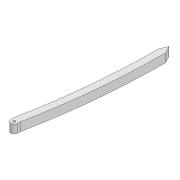
# Autodesk Inventor part: Part_12
Saved by Autodesk Inventor 2022 (Build 260153000, 153)
## iProperties
Created: 2022-05-03
Part Number: Part_12
Material: Generic
Document SubType Name: Modeling
Designer: dell
Density: 1 g/cm^3
Appearance: Default
Author: dell
Autodesk Inventor part; units mm, degrees
ref_plane "YZ Plane" through (0, 0, 0) normal (1, 0, 0) x (0, 1, 0)
ref_plane "XZ Plane" through (0, 0, 0) normal (0, 1, 0) x (-1, 0, 0)
ref_plane "XY Plane" through (0, 0, 0) normal (0, 0, 1) x (1, 0, 0)
sketch "Sketch1" plane through (0, 0, 0) normal (0, 1, 0) x (-1, 0, 0)
  line L0 (0, 0) -> (0, -315.198) construction
  line L1 (-4, 0) -> (-4, -315.198)
  line L2 (4, -315.198) -> (4, 0)
  arc A0 (4, 0) -> (-4, 0) centre (0, 0) ccw
  arc A1 (-4, -315.198) -> (4, -315.198) centre (0, -315.198) ccw
  circle A2 centre (0, 0) radius 1.5
  circle A3 centre (0, -315.198) radius 1.5
  arc A4 (-4, -3) -> (-4, -312.198) centre (780.9198, -157.599) ccw
  arc A5 (4, -3) -> (4, -312.198) centre (788.9198, -157.599) ccw
  point P0 (0, -157.599)
  dimension "d0" = 8
  dimension "d1" = 315.198
  dimension "d2" = 3
  dimension "d3" = 3
  dimension "d24" = 800
  dimension "d25" = 800
  dimension "d26" = 3
  dimension "d27" = 3
  constraints: 8 end point, 8 point on circle, 6 centre point, 4 point on line, 4 tangent, 2 coincident, 2 horizontal alignment, 1 midpoint, 1 parallel, 1 vertical
  measures "d0" diameter of A1
  measures "d1" distance of L0.end L0.start
  measures "d2" diameter of A2
  measures "d3" diameter of A3
  measures "d24" radius of A4
  measures "d25" radius of A5
  measures "d26" vertical distance of L0.end A4.end
  measures "d27" vertical distance of L0.start A4.start
extrude "Extrusion1" add sketch "Sketch1" along normal blind 10 contours A0 L2 A5 L1 | L1 A5 A4 | L1 A5 L2 A1
sketch "Sketch4" plane through (0, 0, 0) normal (0, -1, 0) x (1, 0, 0)
  line L0 (-4, -315.198) -> (-4, -312.198) projected
  arc A0 (-4, -315.198) -> (4, -315.198) centre (0, -315.198) ccw projected
  line L1 (4, -312.198) -> (4, -315.198) projected
  arc A1 (4, -312.198) -> (4, -3) centre (-780.9198, -157.599) ccw projected
  line L2 (4, 0) -> (4, -3) projected
  arc A2 (4, 0) -> (-4, 0) centre (0, 0) ccw projected
  line L3 (-4, -3) -> (-4, 0) projected
  arc A3 (-4, -312.198) -> (-4, -3) centre (-788.9198, -157.599) ccw projected
  circle A4 centre (0, 0) radius 1.5 projected
  circle A5 centre (0, -315.198) radius 1.5 projected
  circle A6 centre (0, -315.198) radius 4
  point P0 (4, -315.198)
  constraints: 1 centre point, 1 coincident, 1 concentric
extrude "Extrusion3" add sketch "Sketch4" along normal blind 10 contours A6 A0
sketch "Sketch3" plane through (0, 10, 0) normal (0, 1, 0) x (1, 0, 0)
  line L0 (-4, 315.198) -> (-4, 312.198) projected
  arc A0 (-4, 3) -> (-4, 312.198) centre (-788.9198, 157.599) ccw projected
  line L1 (-4, 3) -> (-4, 0) projected
  arc A1 (-4, 0) -> (4, 0) centre (0, 0) ccw projected
  line L2 (4, 0) -> (4, 3) projected
  arc A2 (4, 3) -> (4, 312.198) centre (-780.9198, 157.599) ccw projected
  line L3 (4, 312.198) -> (4, 315.198) projected
  arc A3 (4, 315.198) -> (-4, 315.198) centre (0, 315.198) ccw projected
  circle A4 centre (0, 0) radius 1.5 projected
  circle A5 centre (0, 315.198) radius 1.5 projected
  arc A6 (-4, 3) -> (-4, 312.198) centre (-788.9198, 157.599) ccw projected
  line L4 (11.0802, 157.599) -> (14.7286, 165.8884)
  line L5 (14.7286, 165.8884) -> (19.0802, 157.599)
  arc A7 (4, 3) -> (4, 312.198) centre (-780.9198, 157.599) ccw projected
  constraints: 4 end point, 4 point on circle
extrude "Extrusion2" cut sketch "Sketch3" against normal blind 100 contours A3 L3 A2 L5 L4 A0 L0
body "Solid1"
